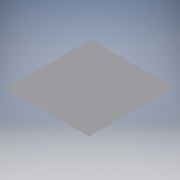
# Autodesk Inventor part: Wand1
Saved by Autodesk Inventor 2018 (Build 220112000, 112)
## iProperties
Created: 2019-02-06
Part Number: Wand1
Material: Generisch
Document SubType Name: Modeling
Designer: Lolob
Density: 1 g/cm^3
Appearance: Vorgabe
Author: Lolob
Autodesk Inventor part; units mm, degrees
ref_plane "YZ Plane" through (0, 0, 0) normal (1, 0, 0) x (0, 1, 0)
ref_plane "XZ Plane" through (0, 0, 0) normal (0, 1, 0) x (-1, 0, 0)
ref_plane "XY Plane" through (0, 0, 0) normal (0, 0, 1) x (1, 0, 0)
sketch "Skizze1" plane through (0, 0, 0) normal (0, 0, 1) x (1, 0, 0)
  line L0 (0, -315) -> (0, 315) projected
  line L1 (-308, 0) -> (308, 0) projected
  line L2 (-220, 225) -> (220, 225)
  line L3 (220, 225) -> (220, -225)
  line L4 (220, -225) -> (-220, -225)
  line L5 (-220, -225) -> (-220, 225)
  point P0 (0, 0)
  dimension "d0" = 440
  dimension "d1" = 450
  constraints: 8 end point, 2 parallel, 1 horizontal, 1 perpendicular, 2 other
  measures "d0" distance of L3.end L4.end
  measures "d1" distance of L4.end L2.start
extrude "Extrusion1" add sketch "Skizze1" along normal blind 20
chamfer "Fase1" distance 20 angle 45 4 edges at (-220, 0, 0) (0, 225, 0) (220, 0, 0) (0, -225, 0)
